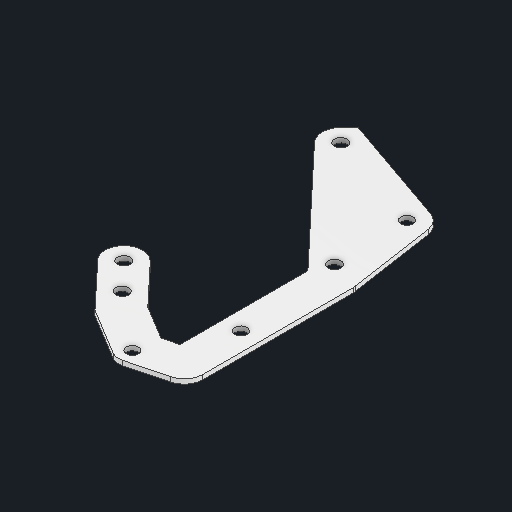
# Autodesk Inventor part: MOGO Funnel
Saved by Autodesk Inventor 2025 (Build 290162000, 162)
## iProperties
Created: 2024-12-27
Part Number: MOGO Funnel
Material: Acetal Resin, White
Document SubType Name: Modeling
Designer: Averey Ku
Density: 1.425 g/cm^3
Appearance: Smooth - White
Author: Averey Ku
Autodesk Inventor part; units mm, degrees
ref_plane "YZ Plane" through (0, 0, 0) normal (1, 0, 0) x (0, 1, 0)
ref_plane "XZ Plane" through (0, 0, 0) normal (0, 1, 0) x (-1, 0, 0)
ref_plane "XY Plane" through (0, 0, 0) normal (0, 0, 1) x (1, 0, 0)
sketch "Sketch1" plane through (0, 0, 0) normal (0, 1, 0) x (-1, 0, 0)
  line L0 (9.4759, 43.9643) -> (23.0237, 29.5342)
  arc A0 (14.5223, 20.0458) -> (23.0237, 29.5342) centre (19.1546, 24.4481) ccw
  line L1 (14.5223, 20.0458) -> (1.4319, 33.9917)
  line L2 (1.4319, 33.9917) -> (-9.9934, 40.8967)
  line L3 (-9.9934, 40.8967) -> (-15.1283, 39.5709)
  line L4 (-6.2902, 53.4927) -> (9.4759, 43.9643)
  arc A1 (-6.2902, 53.4927) -> (-9.9442, 54.0281) centre (-8.7536, 49.4168) ccw
  line L5 (-23.0742, 50.6379) -> (-9.9442, 54.0281)
  arc A2 (-23.0742, 50.6379) -> (-27.8367, 44.4896) centre (-21.4867, 44.4896) ccw
  line L6 (-27.8367, -6.7267) -> (-27.8367, 44.4896)
  line L7 (-15.1283, 39.5709) -> (-15.1283, -3.9855)
  arc A3 (-23.4299, -36.662) -> (-19.226, -41.7322) centre (-17.1484, -35.7317) ccw
  line L8 (-27.7594, -7.429) -> (-23.4299, -36.662)
  circle A4 centre (17.0343, -47.3627) radius 2.1844
  arc A5 (21.39, -51.9834) -> (21.655, -43.007) centre (17.0343, -47.3627) ccw
  line L9 (-15.1283, -3.9855) -> (21.655, -43.007)
  line L10 (21.39, -51.9834) -> (18.4327, -54.771)
  line L11 (-19.226, -41.7322) -> (18.4327, -54.771)
  circle A6 centre (19.1546, 24.4481) radius 2.1844
  circle A7 centre (10.4433, 33.6894) radius 2.1844
  circle A8 centre (-8.7452, 49.4168) radius 2.0955
  circle A9 centre (-17.8109, -10.3972) radius 2.1844
  circle A10 centre (-21.4783, 25.1902) radius 2.0955
  arc A11 (-27.8367, -6.7267) -> (-27.7594, -7.429) centre (-24.6066, -6.7267) ccw
  circle A12 centre (-17.1484, -35.7317) radius 2.0955
  point P0 (0, 0)
  dimension "d0" = 4.191
  dimension "d1" = 4.191
  dimension "d2" = 4.191
  constraints: 24 end point, 13 centre point, 12 point on circle, 4 tangent, 2 coincident, 13 other
  measures "d0" diameter of A8
  measures "d1" diameter of A10
  measures "d2" diameter of A12
extrude "Extrusion1" add sketch "Sketch1" along normal blind 1.5875
body "Solid1"
